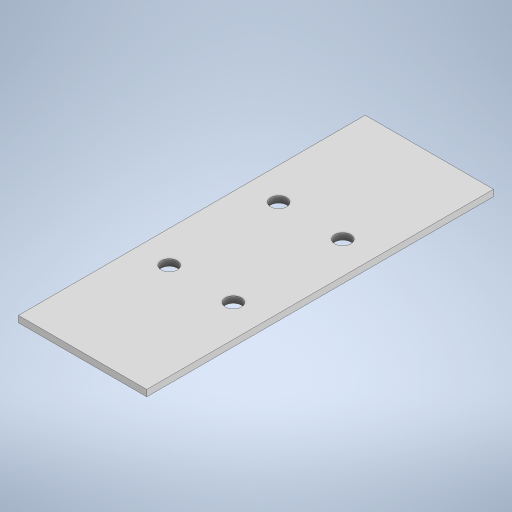
# Autodesk Inventor part: slider_puffer_plate
Saved by Autodesk Inventor 2024 (Build 280153000, 153)
## iProperties
Created: 2025-12-26
Part Number: slider_puffer_plate
Material: Generic
Document SubType Name: Modeling
Designer: schar
Density: 1 g/cm^3
Appearance: Default
Author: schar
Autodesk Inventor part; units mm, degrees
ref_plane "YZ Plane" through (0, 0, 0) normal (1, 0, 0) x (0, 1, 0)
ref_plane "XZ Plane" through (0, 0, 0) normal (0, 1, 0) x (-1, 0, 0)
ref_plane "Work Plane1" through (-20, 3, -54.056) normal (0, 1, 0) x (1, 0, 0)
sketch "Sketch1" plane through (-20, 3, -54.056) normal (0, 1, 0) x (1, 0, 0)
  line L0 (0, 0) -> (0, -108.112) projected
  line L1 (40, -108.112) -> (40, 0) projected
  line L2 (0, 0) -> (40, 0)
  line L3 (40, 0) -> (40, -108.112)
  line L4 (40, -108.112) -> (0, -108.112)
  line L5 (0, -108.112) -> (0, 0)
  circle A0 centre (10, -71.112) radius 2.5 projected
  circle A1 centre (10, -71.112) radius 2.5
  circle A2 centre (30, -71.112) radius 2.5 projected
  circle A3 centre (30, -71.112) radius 2.5
  circle A4 centre (30, -37) radius 2.5 projected
  circle A5 centre (30, -37) radius 2.5
  circle A6 centre (10, -37) radius 2.5 projected
  circle A7 centre (10, -37) radius 2.5
  point P0 (20, -54.056)
  constraints: 8 end point, 4 centre point, 4 coincident, 2 parallel, 1 horizontal, 1 perpendicular
extrude "Extrusion1" add sketch "Sketch1" along normal blind 2
body "Solid1"
